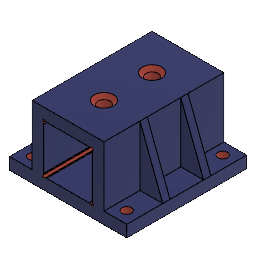
motor mounts v3 (Autodesk Fusion 360 design; units mm, degrees)
Autodesk Fusion 360 part; units mm, degrees
sketch "Sketch1" plane through (0, 0, 0) normal (0, 0, 1) x (1, 0, 0)
  line L0 (0, 0) -> (47, 0)
  line L1 (47, 0) -> (47, 48)
  line L2 (47, 48) -> (0, 48)
  line L3 (0, 48) -> (0, 0)
  circle A0 centre (4, 44) radius 2
  circle A1 centre (4, 4) radius 2
  circle A2 centre (43, 4) radius 2
  circle A3 centre (43, 44) radius 2
  dimension "d1" = 47
  dimension "d2" = 48
  dimension "d102" = 4
  dimension "d103" = 4
  dimension "d104" = 4
  dimension "d105" = 4
  dimension "d114" = 39
  dimension "d115" = 40
  dimension "d116" = 4
  dimension "d117" = 4
  dimension "d118" = 40
  dimension "d119" = 39
  dimension "d120" = 4
  dimension "d121" = 4
  dimension "d122" = 4
  dimension "d123" = 4
  constraint horizontal L0
  constraint vertical L1
  constraint horizontal L2
  constraint vertical L3
  constraint coincident L0.start L3.end
  measures "d1" distance of L0.start L0.end
  measures "d2" distance of L0.start L2.end
  measures "d102" diameter of A0
  measures "d103" diameter of A1
  measures "d104" diameter of A3
  measures "d105" diameter of A2
  measures "d114" distance of A0.centre A3.centre
  measures "d115" distance of A0.centre A1.centre
  measures "d116" distance of L1 A3.centre
  measures "d117" distance of L3 A0.centre
  measures "d118" vertical distance of A2.centre A3.centre
  measures "d119" horizontal distance of A1.centre A2.centre
  measures "d120" distance of L2 A0.centre
  measures "d121" distance of L0 A1.centre
  measures "d122" distance of L2 A3.centre
  measures "d123" distance of L0 A2.centre
extrude "Extrude1" add sketch "Sketch1" along normal blind 3 contours L0 L1 L2 L3 | A0 | A1 | A2 | A3
extrude "Extrude2" add 1 faces at (47, 16, 1) along direction (1, 0, 0) blind 1
extrude "Extrude3" add 1 faces at (16, 0, 1) along direction (0, -1, 0) blind 1
extrude "Extrude4" add 1 faces at (0, 15.3333, 2) along direction (-1, 0, 0) blind 1
extrude "Extrude5" add 1 faces at (31.6667, 48, 1) along direction (0, 1, 0) blind 1
sketch "Sketch2" plane through (0, 0, 3) normal (0, 0, 1) x (-1, 0, 0)
  line L0 (1, 1) -> (-48, 1)
  line L1 (-48, 1) -> (-48, -49)
  line L2 (-48, -49) -> (1, -49)
  line L3 (1, -49) -> (1, 1)
  line L4 (-33.5, -49) -> (-33.5, 1)
  line L5 (-33.5, -49) -> (-13.5, -49)
  line L6 (-13.5, -49) -> (-13.5, 1)
  line L7 (-13.5, 1) -> (-33.5, 1)
  line L8 (-13.5, -49) -> (-8.5, -49)
  line L9 (-8.5, -49) -> (-8.5, 1)
  line L10 (-8.5, 1) -> (-13.5, 1)
  line L11 (-13.5, 1) -> (-13.5, -49)
  line L12 (-33.5, -49) -> (-38.5, -49)
  line L13 (-38.5, -49) -> (-38.5, 1)
  line L14 (-38.5, 1) -> (-33.5, 1)
  line L15 (-33.5, 1) -> (-33.5, -49)
  dimension "d28" = 20
  dimension "d29" = 5
  dimension "d30" = 5
  constraint vertical L4
  constraint horizontal L5
  constraint vertical L6
  constraint horizontal L7
  constraint horizontal L8
  constraint vertical L9
  constraint horizontal L10
  constraint vertical L11
  constraint horizontal L12
  constraint vertical L13
  constraint horizontal L14
  constraint vertical L15
  measures "d28" distance of L4.start L5.end
  measures "d29" distance of L5.end L8.end
  measures "d30" distance of L4.start L12.end
extrude "Extrude6" add sketch "Sketch2" along normal blind 25 contours L0 L2 L4 L12 L13 L14 L15
extrude "Extrude7" add sketch "Sketch2" along normal blind 25 contours L0 L2 L6 L8 L9 L10 L11
sketch "Sketch3" plane through (33.5, 0, 0) normal (-1, 0, 0) x (0, -1, 0)
  line L0 (-49, 3) -> (1, 3)
  line L1 (1, 3) -> (1, 28)
  line L2 (1, 28) -> (-49, 28)
  line L3 (-49, 28) -> (-49, 3)
  line L4 (-49, 28) -> (1, 28)
  line L5 (1, 28) -> (1, 23)
  line L6 (1, 23) -> (-49, 23)
  line L7 (-49, 23) -> (-49, 28)
  dimension "d35" = 5
  constraint horizontal L4
  constraint vertical L5
  constraint horizontal L6
  constraint vertical L7
  constraint coincident L2.end L3.start
  measures "d35" distance of L2.end L6.end
extrude "Extrude8" add sketch "Sketch3" along normal blind 20 contours L1 L2 L3 L4 L5 L6 L7
extrude "Extrude9" add 1 faces at (31.6667, 32.3333, 0) along direction (0, 0, -1) blind 2
sketch "Sketch4" plane through (0, 0, 3) normal (0, 0, 1) x (-1, 0, 0)
  line L0 (-38.5, -49) -> (-38.5, 1)
  line L1 (-38.5, 1) -> (-48, 1)
  line L2 (-48, 1) -> (-48, -49)
  line L3 (-48, -49) -> (-38.5, -49)
  line L4 (-48, 1) -> (-38.5, 1)
  line L5 (-38.5, 1) -> (-38.5, -14)
  line L6 (-38.5, -14) -> (-48, -14)
  line L7 (-48, -14) -> (-48, 1)
  line L8 (-48, -49) -> (-38.5, -49)
  line L9 (-38.5, -49) -> (-38.5, -34)
  line L10 (-38.5, -34) -> (-48, -34)
  line L11 (-48, -34) -> (-48, -49)
  line L12 (-48, -49) -> (-38.5, -49)
  line L13 (-38.5, -49) -> (-38.5, -31)
  line L14 (-38.5, -31) -> (-48, -31)
  line L15 (-48, -31) -> (-48, -49)
  line L16 (-48, 1) -> (-38.5, 1)
  line L17 (-38.5, 1) -> (-38.5, -17)
  line L18 (-38.5, -17) -> (-48, -17)
  line L19 (-48, -17) -> (-48, 1)
  dimension "d40" = 15
  dimension "d41" = 15
  dimension "d42" = 18
  dimension "d43" = 18
  constraint horizontal L4
  constraint vertical L5
  constraint horizontal L6
  constraint vertical L7
  constraint coincident L1.end L2.start
  constraint horizontal L8
  constraint vertical L9
  constraint horizontal L10
  constraint vertical L11
  constraint coincident L2.end L3.start
  constraint horizontal L12
  constraint vertical L13
  constraint horizontal L14
  constraint vertical L15
  constraint horizontal L16
  constraint vertical L17
  constraint horizontal L18
  constraint vertical L19
  measures "d40" distance of L1.end L6.end
  measures "d41" distance of L2.end L10.end
  measures "d42" distance of L2.end L14.end
  measures "d43" distance of L1.end L18.end
extrude "Extrude10" add sketch "Sketch4" along normal blind 25 contours L0 L2 L6 L17 L18 L19
extrude "Extrude11" add sketch "Sketch4" along normal blind 25 contours L0 L2 L10 L13 L14 L15
sketch "Sketch5" plane through (0, 34, 0) normal (0, 1, 0) x (-1, 0, 0)
  line L0 (-48, 3) -> (-38.5, 3)
  line L1 (-38.5, 3) -> (-38.5, 28)
  line L2 (-38.5, 28) -> (-48, 28)
  line L3 (-48, 28) -> (-48, 3)
  line L4 (-38.5, 28) -> (-48, 3)
  constraint coincident L1.end L2.start
  constraint coincident L0.start L3.end
extrude "Extrude12" cut sketch "Sketch5" against normal blind 3 contours L2 L3 L4
sketch "Sketch6" plane through (0, 14, 0) normal (0, -1, 0) x (1, 0, 0)
  line L0 (38.5, 3) -> (48, 3)
  line L1 (48, 3) -> (48, 28)
  line L2 (48, 28) -> (38.5, 28)
  line L3 (38.5, 28) -> (38.5, 3)
  line L4 (38.5, 28) -> (48, 3)
  constraint coincident L2.end L3.start
  constraint coincident L0.end L1.start
extrude "Extrude13" cut sketch "Sketch6" against normal blind 3 contours L1 L2 L4
sketch "Sketch7" plane through (0, 0, 3) normal (0, 0, 1) x (-1, 0, 0)
  line L0 (-8.5, 1) -> (-8.5, -49)
  line L1 (-8.5, -49) -> (1, -49)
  line L2 (1, -49) -> (1, 1)
  line L3 (1, 1) -> (-8.5, 1)
  line L4 (1, -49) -> (-8.5, -49)
  line L5 (-8.5, -49) -> (-8.5, -34)
  line L6 (-8.5, -34) -> (1, -34)
  line L7 (1, -34) -> (1, -49)
  line L8 (1, -34) -> (-8.5, -34)
  line L9 (-8.5, -34) -> (-8.5, -31)
  line L10 (-8.5, -31) -> (1, -31)
  line L11 (1, -31) -> (1, -34)
  line L12 (1, 1) -> (-8.5, 1)
  line L13 (-8.5, 1) -> (-8.5, -14)
  line L14 (-8.5, -14) -> (1, -14)
  line L15 (1, -14) -> (1, 1)
  line L16 (1, -14) -> (-8.5, -14)
  line L17 (-8.5, -14) -> (-8.5, -17)
  line L18 (-8.5, -17) -> (1, -17)
  line L19 (1, -17) -> (1, -14)
  dimension "d52" = 15
  dimension "d53" = 3
  dimension "d54" = 15
  dimension "d55" = 3
  constraint horizontal L4
  constraint vertical L5
  constraint horizontal L6
  constraint vertical L7
  constraint coincident L1.end L2.start
  constraint horizontal L8
  constraint vertical L9
  constraint horizontal L10
  constraint vertical L11
  constraint horizontal L12
  constraint vertical L13
  constraint horizontal L14
  constraint vertical L15
  constraint coincident L2.end L3.start
  constraint horizontal L16
  constraint vertical L17
  constraint horizontal L18
  constraint vertical L19
  measures "d52" distance of L1.end L6.end
  measures "d53" distance of L6.end L10.end
  measures "d54" distance of L2.end L14.end
  measures "d55" distance of L14.end L18.end
extrude "Extrude14" add sketch "Sketch7" along normal blind 25 contours L0 L2 L14 L16 L17 L18 L19 | L0 L2 L6 L8 L9 L10 L11
sketch "Sketch8" plane through (0, 34, 0) normal (0, 1, 0) x (-1, 0, 0)
  line L0 (-8.5, 3) -> (1, 3)
  line L1 (1, 3) -> (1, 28)
  line L2 (1, 28) -> (-8.5, 28)
  line L3 (-8.5, 28) -> (-8.5, 3)
  line L4 (-8.5, 28) -> (1, 3)
  constraint coincident L2.end L3.start
  constraint coincident L0.end L1.start
extrude "Extrude15" cut sketch "Sketch8" against normal blind 3 contours L1 L2 L4
sketch "Sketch9" plane through (0, 17, 0) normal (0, 1, 0) x (-1, 0, 0)
  line L0 (-8.5, 3) -> (1, 3)
  line L1 (1, 3) -> (1, 28)
  line L2 (1, 28) -> (-8.5, 28)
  line L3 (-8.5, 28) -> (-8.5, 3)
  line L4 (-8.5, 28) -> (1, 3)
  constraint coincident L2.end L3.start
  constraint coincident L0.end L1.start
extrude "Extrude16" cut sketch "Sketch9" against normal blind 3 contours L1 L2 L4
move_body "Move1" bodies 1 to x (1, 0, 0) y (0, 1, 0) z (0, 0, 1) at (0, 0, 2)
sketch "Sketch13" plane through (0, -1, 0) normal (0, -1, 0) x (1, 0, 0)
  line L0 (38.5, 30) -> (8.5, 30)
  line L1 (8.5, 30) -> (8.5, 5)
  line L2 (8.5, 5) -> (-1, 5)
  line L3 (-1, 5) -> (-1, 0)
  line L4 (-1, 0) -> (48, 0)
  line L5 (48, 0) -> (48, 5)
  line L6 (48, 5) -> (38.5, 5)
  line L7 (38.5, 5) -> (38.5, 30)
  line L8 (13.5, 25) -> (33.5, 25)
  line L9 (33.5, 25) -> (33.5, 5)
  line L10 (33.5, 5) -> (13.5, 5)
  line L11 (13.5, 5) -> (13.5, 25)
  circle A0 centre (13.5, 25) radius 0.5
  circle A1 centre (33.5, 25) radius 0.5
  circle A2 centre (33.5, 5) radius 0.5
  circle A3 centre (13.5, 5) radius 0.5
  dimension "d74" = 1
  dimension "d75" = 1
  dimension "d76" = 1
  constraint coincident L8.start L11.end
  constraint coincident L8.end L9.start
  constraint coincident L9.end L10.start
  constraint coincident L10.end L11.start
  measures "d74" diameter of A0
  measures "d75" diameter of A2
  measures "d76" diameter of A3
extrude "Extrude20" cut sketch "Sketch13" against normal blind 50 contours L8 L11 A0 | L8 L9 A1 | L10 L11 A3 | L9 L10 A2 picked at (13.1701, 25.0407) picked at (33.402, 25.3176) picked at (13.6495, 4.7031) picked at (33.6442, 4.7005)
fillet "Fillet1" radius 1 8 edges at (33.5, 24, 24.5) (33, 24, 25) (14, 24, 25) (13.5, 24, 24.5) (14, 24, 5) (13.5, 24, 5.5) (33, 24, 5) (33.5, 24, 5.5)
extrude "Extrude21" cut sketch "Sketch1" along normal blind 5 contours A0 | A1 | A2 | A3
sketch "Sketch14" plane through (0, 0, 30) normal (0, 0, 1) x (-1, 0, 0)
  line L0 (-8.5, -17) -> (-8.5, -14)
  line L1 (-8.5, -14) -> (-8.5, 1)
  line L2 (-8.5, 1) -> (-38.5, 1)
  line L3 (-38.5, 1) -> (-38.5, -14)
  line L4 (-38.5, -14) -> (-38.5, -17)
  line L5 (-38.5, -17) -> (-38.5, -31)
  line L6 (-38.5, -31) -> (-38.5, -34)
  line L7 (-38.5, -34) -> (-38.5, -49)
  line L8 (-38.5, -49) -> (-8.5, -49)
  line L9 (-8.5, -49) -> (-8.5, -34)
  line L10 (-8.5, -34) -> (-8.5, -31)
  line L11 (-8.5, -31) -> (-8.5, -17)
  circle A0 centre (-23.5, -34) radius 2.5
  circle A1 centre (-23.5, -14) radius 2.5
hole "Hole1" at (23.5, 34, 30) at (23.5, 14, 30) direction (0, 0, -1) diameter 5 depth 5 tip angle 180 countersink diameter 8 countersink angle 90
extrude "Extrude22" cut 1 faces at (13.5, 32.3333, 12.0393) along direction (-1, 0, 0) blind 0.1
extrude "Extrude23" cut 1 faces at (26.4607, 15.6667, 5) along direction (0, 0, -1) blind 0.1
extrude "Extrude24" cut 1 faces at (33.5, 32.3333, 17.9607) along direction (1, 0, 0) blind 0.1
extrude "Extrude25" cut 1 faces at (23.5, 44.8333, 25) along direction (0, 0, 1) blind 0.1
equation "d121 = d120"
